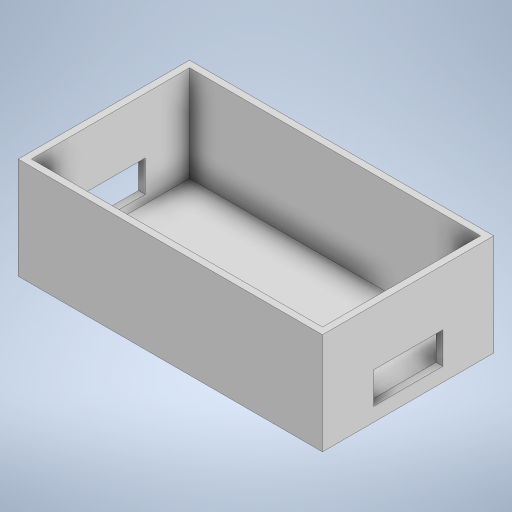
# Autodesk Inventor part: Kenyertarto
Saved by Autodesk Inventor 2023 (Build 270158000, 158)
## iProperties
Created: 2023-04-10
Part Number: Kenyertarto
Material: Generic
Document SubType Name: Modeling
Designer: nagyb
Density: 1 g/cm^3
Appearance: Default
Author: nagyb
Autodesk Inventor part; units mm, degrees
ref_plane "YZ Plane" through (0, 0, 0) normal (1, 0, 0) x (0, 1, 0)
ref_plane "XZ Plane" through (0, 0, 0) normal (0, 1, 0) x (-1, 0, 0)
ref_plane "XY Plane" through (0, 0, 0) normal (0, 0, 1) x (1, 0, 0)
sketch "Sketch1" plane through (0, 0, 0) normal (0, 1, 0) x (-1, 0, 0)
  line L0 (217.5, -122.5) -> (-217.5, -122.5)
  line L1 (-217.5, -122.5) -> (-217.5, 122.5)
  line L2 (-217.5, 122.5) -> (217.5, 122.5)
  line L3 (217.5, 122.5) -> (217.5, -122.5)
  line L4 (217.5, -122.5) -> (-217.5, 122.5) construction
  line L5 (-217.5, -122.5) -> (217.5, 122.5) construction
  point P0 (0, 0)
  dimension "d0" = 435
  dimension "d1" = 245
  constraints: 12 end point, 2 midpoint, 2 parallel, 1 horizontal, 1 perpendicular
  measures "d0" distance of L1.end L2.end
  measures "d1" distance of L2.end L0.start
extrude "Extrusion1" add sketch "Sketch1" along normal blind 145
sketch "Sketch3" plane through (217.5, 0, 122.5) normal (1, 0, 0) x (0, 0, -1)
  line L0 (73, 65) -> (172, 65)
  line L1 (172, 65) -> (172, 20)
  line L2 (172, 20) -> (73, 20)
  line L3 (73, 20) -> (73, 65)
  line L4 (245, 0) -> (245, 145) projected
  line L5 (0, 145) -> (245, 145) projected
  line L6 (0, 5) -> (240, 5) projected
  point P0 (122.5, 0)
  point P1 (172, 42.5)
  dimension "d12" = 73
  dimension "d13" = 80
  dimension "d14" = 99
  dimension "d16" = 45
  constraints: 8 end point, 2 parallel, 1 horizontal, 1 midpoint, 1 perpendicular
  measures "d12" distance from line of L4 point (172, 42.5)
  measures "d13" distance between parallel lines of L5 L0
  measures "d14" distance between parallel lines of L1 L3
  measures "d16" distance of L2.end L0.start
extrude "Extrusion3" cut sketch "Sketch3" against normal blind 450
sketch "Sketch4" plane through (0, 145, 0) normal (0, 1, 0) x (1, 0, 0)
  line L0 (-208, 113) -> (208, 113)
  line L1 (208, 113) -> (208, -113)
  line L2 (208, -113) -> (-208, -113)
  line L3 (-208, -113) -> (-208, 113)
  line L4 (217.5, 122.5) -> (-217.5, 122.5) projected
  line L5 (217.5, -122.5) -> (217.5, 122.5) projected
  line L6 (-217.5, -122.5) -> (217.5, -122.5) projected
  line L7 (-217.5, 122.5) -> (-217.5, -122.5) projected
  point P0 (0, 0)
  dimension "d19" = 9.5
  dimension "d20" = 9.5
  dimension "d21" = 9.5
  dimension "d22" = 9.5
  constraints: 8 end point, 2 parallel, 1 horizontal, 1 perpendicular
  measures "d19" distance between parallel lines of L4 L0
  measures "d20" distance between parallel lines of L5 L1
  measures "d21" distance between parallel lines of L6 L2
  measures "d22" distance between parallel lines of L3 L7
extrude "Extrusion4" cut sketch "Sketch4" against normal blind 137 contours L0 L1 L2 L3
body "Solid1"
